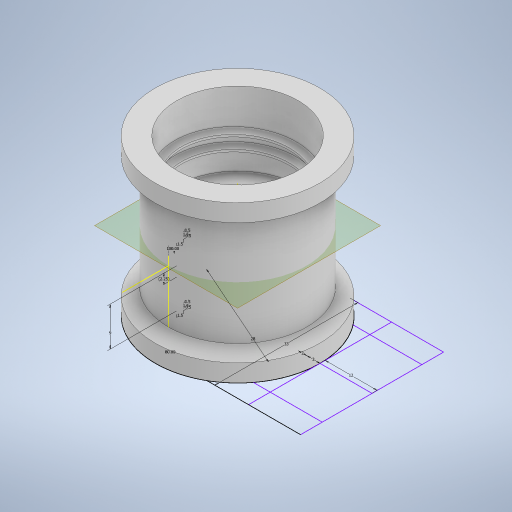
# Autodesk Inventor part: 다단로켓벨브_이음메
Saved by Autodesk Inventor 2023 (Build 270158000, 158)
## iProperties
Created: 2023-08-24
Part Number: 다단로켓벨브_이음메
Material: 일반
Document SubType Name: Modeling
Designer: rlatk
Density: 1 g/cm^3
Appearance: 기본값
Author: rlatk
Autodesk Inventor part; units mm, degrees
ref_plane "YZ Plane" through (0, 0, 0) normal (1, 0, 0) x (0, 1, 0)
ref_plane "XZ Plane" through (0, 0, 0) normal (0, 1, 0) x (-1, 0, 0)
ref_plane "XY Plane" through (0, 0, 0) normal (0, 0, 1) x (1, 0, 0)
sketch "스케치1" plane through (0, 0, 0) normal (0, 1, 0) x (-1, 0, 0)
  circle A0 centre (0, 0) radius 14
  circle A1 centre (0, 0) radius 16
  circle A2 centre (0, 0) radius 19
  line L0 (-9.4207, 16.5) -> (-9.4207, -16.5)
  line L1 (-19, 0) -> (-31, 0)
  line L2 (-9.4207, 16.5) -> (-31, 16.5)
  line L3 (-31, 11.5) -> (-9.4207, 11.5)
  line L4 (-9.4207, 11.5) -> (-9.4207, 16.5)
  line L5 (-9.4207, -16.5) -> (-31, -16.5)
  line L6 (-31, -11.5) -> (-9.4207, -11.5)
  line L7 (-31, 0) -> (-31, 16.5)
  line L8 (-31, 0) -> (-31, -16.5)
  line L9 (-19, -16.5) -> (-19, 16.5)
  point P0 (-15.1245, -11.5)
  point P1 (-15.1245, 11.5)
  point P2 (-9.4207, -11.5)
  point P3 (-9.4207, 11.5)
  point P4 (-19, 11.5)
  point P5 (-19, -11.5)
  dimension "d0" = 28
  dimension "d1" = 2
  dimension "d26" = 3
  dimension "d51" = 33
  dimension "d53" = 12
  constraints: 20 end point, 5 point on line, 3 centre point, 3 point on circle, 2 horizontal, 2 perpendicular, 1 coincident, 1 parallel, 1 symmetric about line, 1 vertical
  measures "d0" diameter of A0
  measures "d1" radial gap between concentric circles of A0 A1
  measures "d26" radial gap between concentric circles of A1 A2
  measures "d51" distance of L0.start L0.end
  measures "d53" distance of L1.start L1.end
extrude "돌출1" add sketch "스케치1" along normal blind 20 contours A0 L0 A1 | A0 L0 L6 A1 L3 | L3 A1 L0 | L0 A1 L6
sketch "스케치2" plane through (0, 0, 0) normal (0, 1, 0) x (-1, 0, 0)
  point P0 (0, 0)
ref_plane "작업 평면1" through (0, 18, 0) normal (0, -1, 0) x (1, 0, 0)
sketch "스케치3" plane through (0, 20, 0) normal (0, 1, 0) x (1, 0, 0)
  point P0 (0, 0)
sketch "스케치4" plane through (0, 18, 0) normal (0, -1, 0) x (1, 0, 0)
  circle A0 centre (0, 0) radius 14 projected
  circle A1 centre (0, 0) radius 14
  circle A2 centre (0, 0) radius 3.85
  dimension "d5" = 7.7
  constraints: 2 centre point, 2 coincident, 1 concentric
  measures "d5" diameter of A2
extrude "돌출2" add sketch "스케치4" along normal blind 1 and the other way blind 1
sketch "스케치5" plane through (0, 0, 0) normal (1, 0, 0) x (0, 1, 0)
  line L0 (17, 14) -> (0, 14) projected
  line L1 (0, 14) -> (0, -14) projected
  line L2 (17, -14) -> (17, 14) projected
  line L3 (17, -14) -> (0, -14) projected
  line L4 (8.75, 14) -> (7.25, 14)
  line L5 (7.25, 14) -> (7.25, 12.5)
  line L6 (7.25, 12.5) -> (8.75, 12.5)
  line L7 (8.75, 12.5) -> (8.75, 14)
  line L8 (8.75, 14) -> (8.25, 12.5)
  line L9 (0, 16) -> (20, 16) projected
  line L10 (0, -16) -> (0, 16) projected
  line L11 (0, -16) -> (20, -16) projected
  line L12 (0, 16) -> (0.3527, 14)
  line L13 (17, 14) -> (0, 14) projected
  line L14 (0, 16) -> (2.0309, 16) construction
  line L15 (0, 16) -> (0, 14)
  line L16 (0.3527, 14) -> (0, 14)
  line L17 (-4.4062, 0) -> (26.437, 0) projected
  line L18 (20, -16) -> (20, 16) projected
  line L19 (20, -16) -> (20, 16) projected
  line L20 (0, -16) -> (0, 16) projected
  line L21 (20, 14) -> (19, 14) projected
  line L22 (20, -14) -> (19, -14) projected
  line L23 (20, 16) -> (20, 14)
  line L24 (20, 16) -> (19.6473, 14)
  line L25 (20, 14) -> (19, 14) projected
  line L26 (20, 16) -> (22.0309, 16) construction
  line L27 (22.1548, 14) -> (22.5074, 14)
  line L28 (20, 13) -> (19, 13) projected
  line L29 (18, -26.6) -> (18, 26.6) projected
  line L30 (0, -16) -> (20, -16) projected
  line L31 (18, -16) -> (18, 16)
  line L32 (0, 16) -> (20, 16) projected
  line L33 (19, 14) -> (19, -14) projected
  line L34 (19, 14) -> (32.2541, 14)
  line L35 (7.75, 12.5) -> (7.25, 14)
  line L36 (23.0074, 14) -> (21.5074, 14)
  line L37 (21.5074, 14) -> (21.5074, 12.5)
  line L38 (21.5074, 12.5) -> (23.0074, 12.5)
  line L39 (23.0074, 12.5) -> (23.0074, 14)
  line L40 (23.0074, 14) -> (22.5074, 12.5)
  line L41 (22.0074, 12.5) -> (21.5074, 14)
  point P0 (0, 0)
  point P1 (8.75, 13.25)
  point P2 (8, 14)
  point P3 (7.25, 13.9506)
  dimension "d10" = 1.5
  dimension "d11" = 1.5
  dimension "d13" = 9
  dimension "d14" = 0.5
  dimension "d15" = 0.5
  dimension "d24" = 80
  dimension "d32" = 100
  dimension "d95" = 1.5
  dimension "d96" = 1.5
  dimension "d97" = 0.5
  dimension "d98" = 0.5
  constraints: 44 end point, 11 point on line, 6 horizontal, 4 parallel, 2 collinear, 2 equal length, 2 midpoint, 2 perpendicular, 1 vertical, 2 other
  measures "d10" distance of L6.end L5.end
  measures "d11" distance of L5.end L4.end
  measures "d13" distance from line of L2 point (8, 14)
  measures "d14" distance of L8.end L6.end
  measures "d15" distance of L5.end L35.start
  measures "d24" angle of L12 L14
  measures "d32" angle of L24 L26
  measures "d95" distance of L38.end L38.start
  measures "d96" distance of L38.start L41.end
  measures "d97" distance of L40.end L38.end
  measures "d98" distance of L38.start L41.start
coil "코일1" sketch "스케치5" operation add axis through (0, -10, 0) along (0, 1, 0) pitch 3 turns 2 hand right contours L8 L6 L35 L0
revolve "회전1" cut sketch "스케치5" angle 360 about axis through (0, -10, 0) along (0, 1, 0) contours L0 L10 L12
extrude "돌출3" add sketch "스케치1" along normal blind 4 contours L0 A2 A1 | A1 L3 A2 L0 | A1 L6 A2 L3 | L0 A2 L6 A1
sketch "스케치6" plane through (0, 0, 0) normal (1, 0, 0) x (0, 1, 0)
  line L0 (4, -19) -> (4, 19) projected
  line L1 (4, 19) -> (5.7321, 16)
  line L2 (4, 16) -> (20, 16) projected
  line L3 (4, 19) -> (7.4641, 19) construction
  line L4 (5.7321, 16) -> (4, 16)
  line L5 (4, 16) -> (4, 19)
  line L6 (-4, 0) -> (24, 0) projected
  point P0 (0, 0)
  dimension "d29" = 60
  constraints: 8 end point, 2 point on line, 1 equal length, 1 horizontal, 1 perpendicular
  measures "d29" angle of L1 L3
revolve "회전2" add sketch "스케치6" angle 360 about axis through (0, -10, 0) along (0, 1, 0)
mirror "미러5" about plane through (0, 18, 0) normal (0, -1, 0) of "돌출3", "회전2", "돌출1"
sketch "스케치17" plane through (0, 0, 0) normal (1, 0, 0) x (0, 1, 0)
  line L0 (8.25, 12.5) -> (8.75, 14) projected
  line L1 (14.25, 12.5) -> (14.75, 14) projected
  line L2 (17, -14) -> (17, 14) projected
  point P0 (0, 0)
  dimension "d99" = 2.25
  constraints: 2 horizontal alignment
  measures "d99" distance from line of L1.end L2
coil "코일2" sketch "스케치5" operation add axis through (0, -10, 0) along (0, 1, 0) pitch 3 turns 2 hand right contours L27 L34 L40 L38 L41
